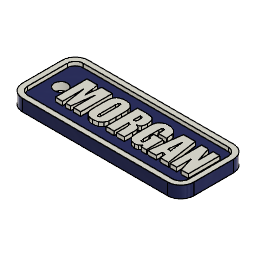
Mini Keychain (Autodesk Fusion 360 design; units mm, degrees)
part number: 2025-11-17-21-09-36-714
Autodesk Fusion 360 part; units mm, degrees
sketch "Sketch1" plane through (0, 0, 0) normal (0, 0, 1) x (1, 0, 0)
  line L0 (-5, 0) -> (-60, 0)
  line L1 (-65, 5) -> (-65, 20)
  line L2 (-60, 25) -> (-5, 25)
  line L3 (0, 20) -> (0, 5)
  arc A0 (0, 20) -> (-5, 25) centre (-5, 20) ccw
  arc A1 (-5, 0) -> (0, 5) centre (-5, 5) ccw
  arc A2 (-65, 5) -> (-60, 0) centre (-60, 5) ccw
  arc A3 (-60, 25) -> (-65, 20) centre (-60, 20) ccw
  line L4 (-5, 2) -> (-60, 2)
  arc A4 (-63, 5) -> (-60, 2) centre (-60, 5) ccw
  line L5 (-63, 5) -> (-63, 20)
  arc A5 (-60, 23) -> (-63, 20) centre (-60, 20) ccw
  line L6 (-60, 23) -> (-5, 23)
  arc A6 (-2, 20) -> (-5, 23) centre (-5, 20) ccw
  line L7 (-2, 20) -> (-2, 5)
  arc A7 (-5, 2) -> (-2, 5) centre (-5, 5) ccw
  line L8 (-58, 25) -> (-58, 0) construction
  circle A8 centre (-58, 12.5) radius 2.5
  line L9 (-52.9506, 5.1049) -> (-4.9506, 5.1049) construction
  line L10 (-4.9506, 5.1049) -> (-4.9506, 20.1049) construction
  line L11 (-4.9506, 20.1049) -> (-52.9506, 20.1049) construction
  line L12 (-52.9506, 20.1049) -> (-52.9506, 5.1049) construction
  point P0 (-65, 0)
  point P1 (0, 25)
  point P2 (-58, 12.5)
  dimension "d1" = 65
  dimension "d2" = 25
  dimension "d3" = 2
  dimension "d4" = 5
  dimension "d5" = 7
  dimension "d6" = 5
  dimension "d7" = 12
  text T0 "MORGAN" font "Impact" height 12 align centre middle in box 48 x 15 at (-52.9506, 5.1049) x (1, 0) y (0, 1) spacing 1
  constraint horizontal L0
  constraint vertical L1
  constraint horizontal L2
  constraint vertical L3
  constraint coincident P1 L2
  constraint coincident P1 L3
  constraint tangent L2 A0
  constraint tangent L3 A0
  constraint coincident origin L0
  constraint coincident origin L3
  constraint tangent L0 A1
  constraint tangent L3 A1
  constraint equal A0 A1
  constraint coincident P0 L0
  constraint coincident P0 L1
  constraint tangent L0 A2
  constraint tangent L1 A2
  constraint equal A0 A2
  constraint tangent L1 A3
  constraint tangent L2 A3
  constraint equal A0 A3
  constraint coincident L2 L8.start
  constraint coincident L0 L8.end
  constraint perpendicular L0 L8
  constraint midpoint L8 P2
  constraint coincident P2 A8.centre
  measures "d1" distance of origin P0
  measures "d2" distance of origin P1
  measures "d4" radius of A0
  measures "d5" distance of L1 L8
  measures "d6" diameter of A8
extrude "Extrude1" add sketch "Sketch1" along normal blind 3 contours L0 L1 L2 L3 A0 A1 A2 A3 | L4 A4 L5 A5 L6 A6 L7 A7
extrude "Extrude2" add sketch "Sketch1" sketch "Sketch1" along normal blind 1.5 from surface at 3 contours L0 L1 L2 L3 A0 A1 A2 A3 of sketch 2 text T0
equation "d8 = 'MORGAN'"
